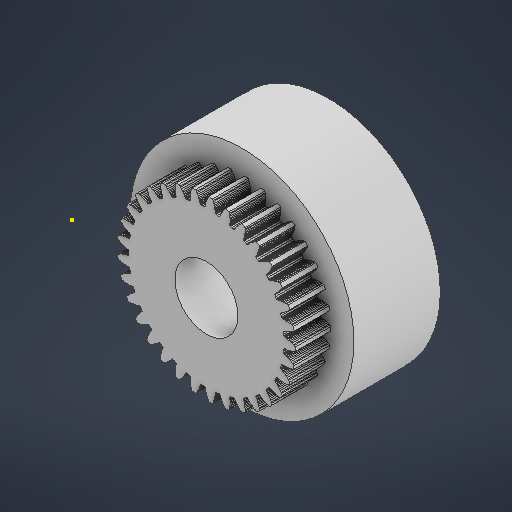
# Autodesk Inventor part: EngranajeRueda
Saved by Autodesk Inventor 2027 (Build 310192060, 192F)
## iProperties
Created: 2026-08-10
Part Number: EngranajeRueda
Material: Generic
Document SubType Name: Modeling
Designer: Administrator
Density: 1 g/cm^3
Appearance: Default
Author: Administrator
Autodesk Inventor part; units mm, degrees
(part 1 of 3)
ref_plane "YZ Plane" through (0, 0, 0) normal (1, 0, 0) x (0, 1, 0)
ref_plane "XZ Plane" through (0, 0, 0) normal (0, 1, 0) x (-1, 0, 0)
ref_plane "XY Plane" through (0, 0, 0) normal (0, 0, 1) x (1, 0, 0)
sketch "Sketch1" plane through (0, 0, 0) normal (0, 0, 1) x (1, 0, 0)
  point P0 (0, 0)
sketch "Sketch2" plane through (0, 0, 0) normal (0, 0, 1) x (1, 0, 0)
  circle A0 centre (13.25, 0) radius 4
  circle A1 centre (13.25, 0) radius 4
  line L0 (0, -0.275) -> (0, 0.275)
  line L1 (-0.275, 0) -> (0.275, 0)
  line L2 (0, -0.275) -> (0, 0.275)
  line L3 (-0.275, 0) -> (0.275, 0)
  line L4 (4.9115, -2.1897) -> (4.9704, -2.1401)
  line L5 (4.9704, -2.1401) -> (5.0843, -2.0503)
  line L6 (5.0843, -2.0503) -> (5.1901, -1.9738)
  line L7 (5.1901, -1.9738) -> (5.2873, -1.9095)
  line L8 (5.2873, -1.9095) -> (5.3762, -1.8559)
  line L9 (5.3762, -1.8559) -> (5.4548, -1.8129)
  line L10 (5.4548, -1.8129) -> (5.5252, -1.7781)
  line L11 (5.5252, -1.7781) -> (5.5804, -1.7537)
  line L12 (5.5804, -1.7537) -> (5.6607, -1.7208)
  line L13 (5.6607, -1.7208) -> (5.6881, -1.7069)
  line L14 (5.6881, -1.7069) -> (5.7116, -1.6927)
  line L15 (5.7116, -1.6927) -> (5.7313, -1.6783)
  line L16 (5.7313, -1.6783) -> (5.747, -1.6639)
  line L17 (5.747, -1.6639) -> (5.7588, -1.6496)
  line L18 (5.7588, -1.6496) -> (5.7667, -1.6357)
  line L19 (5.7667, -1.6357) -> (5.7708, -1.6222)
  line L20 (5.7708, -1.6222) -> (5.7711, -1.6094)
  line L21 (5.7711, -1.6094) -> (5.7661, -1.5858)
  line L22 (5.7661, -1.5858) -> (5.7382, -1.4478)
  line L23 (5.7382, -1.4478) -> (5.7128, -1.3093)
  line L24 (5.7128, -1.3093) -> (5.7087, -1.2856)
  line L25 (5.7087, -1.2856) -> (5.7036, -1.2737)
  line L26 (5.7036, -1.2737) -> (5.6948, -1.2627)
  line L27 (5.6948, -1.2627) -> (5.6823, -1.2527)
  line L28 (5.6823, -1.2527) -> (5.666, -1.2439)
  line L29 (5.666, -1.2439) -> (5.6461, -1.2364)
  line L30 (5.6461, -1.2364) -> (5.6225, -1.2303)
  line L31 (5.6225, -1.2303) -> (5.5954, -1.2258)
  line L32 (5.5954, -1.2258) -> (5.5648, -1.2231)
  line L33 (5.5648, -1.2231) -> (5.478, -1.2224)
  line L34 (5.478, -1.2224) -> (5.4177, -1.2203)
  line L35 (5.4177, -1.2203) -> (5.3394, -1.2142)
  line L36 (5.3394, -1.2142) -> (5.2505, -1.2034)
  line L37 (5.2505, -1.2034) -> (5.148, -1.1867)
  line L38 (5.148, -1.1867) -> (5.0338, -1.1631)
  line L39 (5.0338, -1.1631) -> (4.9072, -1.1315)
  line L40 (4.9072, -1.1315) -> (4.7681, -1.0904)
  line L41 (4.7681, -1.0904) -> (4.695, -1.0663)
  line L42 (4.695, -1.0663) -> (4.5593, -1.0171)
  arc A2 (4.5239, -0.646) -> (4.5593, -1.0171) centre (13.25, 0) ccw
  line L43 (4.5239, -0.646) -> (4.6478, -0.572)
  line L44 (4.6478, -0.572) -> (4.715, -0.5346)
  line L45 (4.715, -0.5346) -> (4.8439, -0.4679)
  line L46 (4.8439, -0.4679) -> (4.9622, -0.4128)
  line L47 (4.9622, -0.4128) -> (5.0698, -0.368)
  line L48 (5.0698, -0.368) -> (5.1673, -0.3322)
  line L49 (5.1673, -0.3322) -> (5.2526, -0.3049)
  line L50 (5.2526, -0.3049) -> (5.3283, -0.2841)
  line L51 (5.3283, -0.2841) -> (5.3871, -0.2705)
  line L52 (5.3871, -0.2705) -> (5.4722, -0.2535)
  line L53 (5.4722, -0.2535) -> (5.5017, -0.245)
  line L54 (5.5017, -0.245) -> (5.5275, -0.2354)
  line L55 (5.5275, -0.2354) -> (5.5495, -0.225)
  line L56 (5.5495, -0.225) -> (5.5677, -0.2139)
  line L57 (5.5677, -0.2139) -> (5.582, -0.2021)
  line L58 (5.582, -0.2021) -> (5.5924, -0.1899)
  line L59 (5.5924, -0.1899) -> (5.599, -0.1775)
  line L60 (5.599, -0.1775) -> (5.6017, -0.1649)
  line L61 (5.6017, -0.1649) -> (5.6013, -0.1408)
  line L62 (5.6013, -0.1408) -> (5.6, 0)
  line L63 (5.6, 0) -> (5.6013, 0.1408)
  line L64 (5.6013, 0.1408) -> (5.6017, 0.1649)
  line L65 (5.6017, 0.1649) -> (5.599, 0.1775)
  line L66 (5.599, 0.1775) -> (5.5924, 0.1899)
  line L67 (5.5924, 0.1899) -> (5.582, 0.2021)
  line L68 (5.582, 0.2021) -> (5.5677, 0.2139)
  line L69 (5.5677, 0.2139) -> (5.5495, 0.225)
  line L70 (5.5495, 0.225) -> (5.5275, 0.2354)
  line L71 (5.5275, 0.2354) -> (5.5017, 0.245)
  line L72 (5.5017, 0.245) -> (5.4722, 0.2535)
  line L73 (5.4722, 0.2535) -> (5.3871, 0.2705)
  line L74 (5.3871, 0.2705) -> (5.3283, 0.2841)
  line L75 (5.3283, 0.2841) -> (5.2526, 0.3049)
  line L76 (5.2526, 0.3049) -> (5.1673, 0.3322)
  line L77 (5.1673, 0.3322) -> (5.0698, 0.368)
  line L78 (5.0698, 0.368) -> (4.9622, 0.4128)
  line L79 (4.9622, 0.4128) -> (4.8439, 0.4679)
  line L80 (4.8439, 0.4679) -> (4.715, 0.5346)
  line L81 (4.715, 0.5346) -> (4.6478, 0.572)
  line L82 (4.6478, 0.572) -> (4.5239, 0.646)
  arc A3 (4.5593, 1.0171) -> (4.5239, 0.646) centre (13.25, 0) ccw
  line L83 (4.5593, 1.0171) -> (4.695, 1.0663)
  line L84 (4.695, 1.0663) -> (4.7681, 1.0904)
  line L85 (4.7681, 1.0904) -> (4.9072, 1.1315)
  line L86 (4.9072, 1.1315) -> (5.0338, 1.1631)
  line L87 (5.0338, 1.1631) -> (5.148, 1.1867)
  line L88 (5.148, 1.1867) -> (5.2505, 1.2034)
  line L89 (5.2505, 1.2034) -> (5.3394, 1.2142)
  line L90 (5.3394, 1.2142) -> (5.4177, 1.2203)
  line L91 (5.4177, 1.2203) -> (5.478, 1.2224)
  line L92 (5.478, 1.2224) -> (5.5648, 1.2231)
  line L93 (5.5648, 1.2231) -> (5.5954, 1.2258)
  line L94 (5.5954, 1.2258) -> (5.6225, 1.2303)
  line L95 (5.6225, 1.2303) -> (5.6461, 1.2364)
  line L96 (5.6461, 1.2364) -> (5.666, 1.2439)
  line L97 (5.666, 1.2439) -> (5.6823, 1.2527)
  line L98 (5.6823, 1.2527) -> (5.6948, 1.2627)
  line L99 (5.6948, 1.2627) -> (5.7036, 1.2737)
  line L100 (5.7036, 1.2737) -> (5.7087, 1.2856)
  line L101 (5.7087, 1.2856) -> (5.7128, 1.3093)
  line L102 (5.7128, 1.3093) -> (5.7382, 1.4478)
  line L103 (5.7382, 1.4478) -> (5.7661, 1.5858)
  line L104 (5.7661, 1.5858) -> (5.7711, 1.6094)
  line L105 (5.7711, 1.6094) -> (5.7708, 1.6222)
  line L106 (5.7708, 1.6222) -> (5.7667, 1.6357)
  line L107 (5.7667, 1.6357) -> (5.7588, 1.6496)
  line L108 (5.7588, 1.6496) -> (5.747, 1.6639)
  line L109 (5.747, 1.6639) -> (5.7313, 1.6783)
  line L110 (5.7313, 1.6783) -> (5.7116, 1.6927)
  line L111 (5.7116, 1.6927) -> (5.6881, 1.7069)
  line L112 (5.6881, 1.7069) -> (5.6607, 1.7208)
  line L113 (5.6607, 1.7208) -> (5.5804, 1.7537)
  line L114 (5.5804, 1.7537) -> (5.5252, 1.7781)
  line L115 (5.5252, 1.7781) -> (5.4548, 1.8129)
  line L116 (5.4548, 1.8129) -> (5.3762, 1.8559)
  line L117 (5.3762, 1.8559) -> (5.2873, 1.9095)
  line L118 (5.2873, 1.9095) -> (5.1901, 1.9738)
  line L119 (5.1901, 1.9738) -> (5.0843, 2.0503)
  line L120 (5.0843, 2.0503) -> (4.9704, 2.1401)
  line L121 (4.9704, 2.1401) -> (4.9115, 2.1897)
  line L122 (4.9115, 2.1897) -> (4.8038, 2.2858)
  arc A4 (4.9089, 2.6434) -> (4.8038, 2.2858) centre (13.25, 0) ccw
  line L123 (4.9089, 2.6434) -> (5.0514, 2.666)
  line L124 (5.0514, 2.666) -> (5.1277, 2.6759)
  line L125 (5.1277, 2.6759) -> (5.2721, 2.6899)
  line L126 (5.2721, 2.6899) -> (5.4024, 2.697)
  line L127 (5.4024, 2.697) -> (5.519, 2.6986)
  line L128 (5.519, 2.6986) -> (5.6228, 2.6956)
  line L129 (5.6228, 2.6956) -> (5.7121, 2.6893)
  line L130 (5.7121, 2.6893) -> (5.7902, 2.6805)
  line L131 (5.7902, 2.6805) -> (5.8498, 2.6712)
  line L132 (5.8498, 2.6712) -> (5.9351, 2.6554)
  line L133 (5.9351, 2.6554) -> (5.9657, 2.6523)
  line L134 (5.9657, 2.6523) -> (5.9932, 2.6516)
  line L135 (5.9932, 2.6516) -> (6.0175, 2.6531)
  line L136 (6.0175, 2.6531) -> (6.0385, 2.6567)
  line L137 (6.0385, 2.6567) -> (6.0561, 2.6623)
  line L138 (6.0561, 2.6623) -> (6.0703, 2.6697)
  line L139 (6.0703, 2.6697) -> (6.0811, 2.6789)
  line L140 (6.0811, 2.6789) -> (6.0882, 2.6895)
  line L141 (6.0882, 2.6895) -> (6.0968, 2.712)
  line L142 (6.0968, 2.712) -> (6.148, 2.8432)
  line L143 (6.148, 2.8432) -> (6.2015, 2.9735)
  line L144 (6.2015, 2.9735) -> (6.2108, 2.9957)
  line L145 (6.2108, 2.9957) -> (6.213, 3.0083)
  line L146 (6.213, 3.0083) -> (6.2115, 3.0223)
  line L147 (6.2115, 3.0223) -> (6.2064, 3.0375)
  line L148 (6.2064, 3.0375) -> (6.1974, 3.0538)
  line L149 (6.1974, 3.0538) -> (6.1847, 3.0709)
  line L150 (6.1847, 3.0709) -> (6.1682, 3.0887)
  line L151 (6.1682, 3.0887) -> (6.1478, 3.1072)
  line L152 (6.1478, 3.1072) -> (6.1235, 3.126)
  line L153 (6.1235, 3.126) -> (6.0508, 3.1735)
  line L154 (6.0508, 3.1735) -> (6.0013, 3.2079)
  line L155 (6.0013, 3.2079) -> (5.9387, 3.2554)
  line L156 (5.9387, 3.2554) -> (5.8698, 3.3125)
  line L157 (5.8698, 3.3125) -> (5.7926, 3.3819)
  line L158 (5.7926, 3.3819) -> (5.7093, 3.4635)
  line L159 (5.7093, 3.4635) -> (5.6199, 3.5586)
  line L160 (5.6199, 3.5586) -> (5.5251, 3.6684)
  line L161 (5.5251, 3.6684) -> (5.4766, 3.7282)
  line L162 (5.4766, 3.7282) -> (5.3891, 3.8429)
  arc A5 (5.5599, 4.1742) -> (5.3891, 3.8429) centre (13.25, 0) ccw
  line L163 (5.5599, 4.1742) -> (5.7041, 4.1695)
  line L164 (5.7041, 4.1695) -> (5.7809, 4.1647)
  line L165 (5.7809, 4.1647) -> (5.9254, 4.1511)
  line L166 (5.9254, 4.1511) -> (6.0547, 4.1335)
  line L167 (6.0547, 4.1335) -> (6.1694, 4.1129)
  line L168 (6.1694, 4.1129) -> (6.2708, 4.0904)
  line L169 (6.2708, 4.0904) -> (6.3573, 4.0673)
  line L170 (6.3573, 4.0673) -> (6.4323, 4.0438)
  line L171 (6.4323, 4.0438) -> (6.489, 4.0235)
  line L172 (6.489, 4.0235) -> (6.5698, 3.9918)
  line L173 (6.5698, 3.9918) -> (6.5993, 3.9829)
  line L174 (6.5993, 3.9829) -> (6.6262, 3.977)
  line L175 (6.6262, 3.977) -> (6.6503, 3.9739)
  line L176 (6.6503, 3.9739) -> (6.6716, 3.9735)
  line L177 (6.6716, 3.9735) -> (6.69, 3.9756)
  line L178 (6.69, 3.9756) -> (6.7053, 3.9802)
  line L179 (6.7053, 3.9802) -> (6.7176, 3.9872)
  line L180 (6.7176, 3.9872) -> (6.7267, 3.9963)
  line L181 (6.7267, 3.9963) -> (6.7394, 4.0168)
  line L182 (6.7394, 4.0168) -> (6.8144, 4.1359)
  line L183 (6.8144, 4.1359) -> (6.8916, 4.2537)
  line L184 (6.8916, 4.2537) -> (6.9049, 4.2737)
  line L185 (6.9049, 4.2737) -> (6.9095, 4.2857)
  line L186 (6.9095, 4.2857) -> (6.9107, 4.2998)
  line L187 (6.9107, 4.2998) -> (6.9085, 4.3157)
  line L188 (6.9085, 4.3157) -> (6.9028, 4.3333)
  line L189 (6.9028, 4.3333) -> (6.8936, 4.3525)
  line L190 (6.8936, 4.3525) -> (6.8807, 4.3732)
  line L191 (6.8807, 4.3732) -> (6.8642, 4.3951)
  line L192 (6.8642, 4.3951) -> (6.8439, 4.4182)
  line L193 (6.8439, 4.4182) -> (6.7815, 4.4786)
  line L194 (6.7815, 4.4786) -> (6.7394, 4.5218)
  line L195 (6.7394, 4.5218) -> (6.6869, 4.5802)
  line L196 (6.6869, 4.5802) -> (6.63, 4.6493)
  line L197 (6.63, 4.6493) -> (6.5674, 4.7321)
  line L198 (6.5674, 4.7321) -> (6.501, 4.828)
  line L199 (6.501, 4.828) -> (6.4313, 4.9383)
  line L200 (6.4313, 4.9383) -> (6.3589, 5.064)
  line L201 (6.3589, 5.064) -> (6.3226, 5.1319)
  line L202 (6.3226, 5.1319) -> (6.2584, 5.2612)
  arc A6 (6.4888, 5.5542) -> (6.2584, 5.2612) centre (13.25, 0) ccw
  line L203 (6.4888, 5.5542) -> (6.6295, 5.5222)
  line L204 (6.6295, 5.5222) -> (6.7041, 5.5029)
  line L205 (6.7041, 5.5029) -> (6.8433, 5.4623)
  line L206 (6.8433, 5.4623) -> (6.967, 5.4205)
  line L207 (6.967, 5.4205) -> (7.0758, 5.3786)
  line L208 (7.0758, 5.3786) -> (7.171, 5.3373)
  line L209 (7.171, 5.3373) -> (7.2516, 5.2982)
  line L210 (7.2516, 5.2982) -> (7.3208, 5.261)
  line L211 (7.3208, 5.261) -> (7.3727, 5.2303)
  line L212 (7.3727, 5.2303) -> (7.446, 5.1839)
  line L213 (7.446, 5.1839) -> (7.4733, 5.1696)
  line L214 (7.4733, 5.1696) -> (7.4985, 5.1587)
  line L215 (7.4985, 5.1587) -> (7.5216, 5.1511)
  line L216 (7.5216, 5.1511) -> (7.5424, 5.1466)
  line L217 (7.5424, 5.1466) -> (7.5609, 5.1453)
  line L218 (7.5609, 5.1453) -> (7.5769, 5.1469)
  line L219 (7.5769, 5.1469) -> (7.5902, 5.1514)
  line L220 (7.5902, 5.1514) -> (7.6008, 5.1586)
  line L221 (7.6008, 5.1586) -> (7.6172, 5.1763)
  line L222 (7.6172, 5.1763) -> (7.7134, 5.2791)
  line L223 (7.7134, 5.2791) -> (7.8115, 5.3801)
  line L224 (7.8115, 5.3801) -> (7.8284, 5.3973)
  line L225 (7.8284, 5.3973) -> (7.8352, 5.4082)
  line L226 (7.8352, 5.4082) -> (7.839, 5.4218)
  line L227 (7.839, 5.4218) -> (7.8399, 5.4378)
  line L228 (7.8399, 5.4378) -> (7.8376, 5.4562)
  line L229 (7.8376, 5.4562) -> (7.8322, 5.4768)
  line L230 (7.8322, 5.4768) -> (7.8235, 5.4995)
  line L231 (7.8235, 5.4995) -> (7.8114, 5.5242)
  line L232 (7.8114, 5.5242) -> (7.7958, 5.5508)
  line L233 (7.7958, 5.5508) -> (7.746, 5.6218)
  line L234 (7.746, 5.6218) -> (7.7128, 5.6722)
  line L235 (7.7128, 5.6722) -> (7.6724, 5.7395)
  line L236 (7.6724, 5.7395) -> (7.6295, 5.8181)
  line L237 (7.6295, 5.8181) -> (7.5837, 5.9113)
  line L238 (7.5837, 5.9113) -> (7.5367, 6.018)
  line L239 (7.5367, 6.018) -> (7.4891, 6.1395)
  line L240 (7.4891, 6.1395) -> (7.4418, 6.2767)
  line L241 (7.4418, 6.2767) -> (7.4191, 6.3502)
  line L242 (7.4191, 6.3502) -> (7.3804, 6.4893)
  arc A7 (7.6621, 6.7334) -> (7.3804, 6.4893) centre (13.25, 0) ccw
  line L243 (7.6621, 6.7334) -> (7.7943, 6.6753)
  line L244 (7.7943, 6.6753) -> (7.8638, 6.6423)
  line L245 (7.8638, 6.6423) -> (7.9928, 6.576)
  line L246 (7.9928, 6.576) -> (8.1063, 6.5116)
  line L247 (8.1063, 6.5116) -> (8.2052, 6.4499)
  line L248 (8.2052, 6.4499) -> (8.291, 6.3913)
  line L249 (8.291, 6.3913) -> (8.3627, 6.3377)
  line L250 (8.3627, 6.3377) -> (8.4236, 6.2881)
  line L251 (8.4236, 6.2881) -> (8.4687, 6.248)
  line L252 (8.4687, 6.248) -> (8.532, 6.1886)
  line L253 (8.532, 6.1886) -> (8.556, 6.1694)
  line L254 (8.556, 6.1694) -> (8.5787, 6.154)
  line L255 (8.5787, 6.154) -> (8.6, 6.1421)
  line L256 (8.6, 6.1421) -> (8.6196, 6.1338)
  line L257 (8.6196, 6.1338) -> (8.6375, 6.129)
  line L258 (8.6375, 6.129) -> (8.6535, 6.1275)
  line L259 (8.6535, 6.1275) -> (8.6674, 6.1294)
  line L260 (8.6674, 6.1294) -> (8.6792, 6.1345)
  line L261 (8.6792, 6.1345) -> (8.6986, 6.1488)
  line L262 (8.6986, 6.1488) -> (8.8126, 6.2315)
  line L263 (8.8126, 6.2315) -> (8.928, 6.3121)
  line L264 (8.928, 6.3121) -> (8.9478, 6.3258)
  line L265 (8.9478, 6.3258) -> (8.9565, 6.3353)
  line L266 (8.9565, 6.3353) -> (8.9629, 6.3479)
  line L267 (8.9629, 6.3479) -> (8.9667, 6.3634)
  line L268 (8.9667, 6.3634) -> (8.968, 6.3819)
  line L269 (8.968, 6.3819) -> (8.9666, 6.4032)
  line L270 (8.9666, 6.4032) -> (8.9623, 6.4271)
  line L271 (8.9623, 6.4271) -> (8.9551, 6.4536)
  line L272 (8.9551, 6.4536) -> (8.9449, 6.4827)
  line L273 (8.9449, 6.4827) -> (8.9094, 6.5619)
  line L274 (8.9094, 6.5619) -> (8.8863, 6.6176)
  line L275 (8.8863, 6.6176) -> (8.8594, 6.6914)
  line L276 (8.8594, 6.6914) -> (8.8322, 6.7767)
  line L277 (8.8322, 6.7767) -> (8.8048, 6.8769)
  line L278 (8.8048, 6.8769) -> (8.7788, 6.9905)
  line L279 (8.7788, 6.9905) -> (8.7551, 7.1188)
  line L280 (8.7551, 7.1188) -> (8.7347, 7.2624)
  line L281 (8.7347, 7.2624) -> (8.7262, 7.339)
  line L282 (8.7262, 7.339) -> (8.7146, 7.4828)
  arc A8 (9.0374, 7.6692) -> (8.7146, 7.4828) centre (13.25, 0) ccw
  line L283 (9.0374, 7.6692) -> (9.1562, 7.5872)
  line L284 (9.1562, 7.5872) -> (9.2182, 7.5416)
  line L285 (9.2182, 7.5416) -> (9.3324, 7.4521)
  line L286 (9.3324, 7.4521) -> (9.4316, 7.3674)
  line L287 (9.4316, 7.3674) -> (9.5171, 7.2881)
  line L288 (9.5171, 7.2881) -> (9.5901, 7.2143)
  line L289 (9.5901, 7.2143) -> (9.6504, 7.1481)
  line L290 (9.6504, 7.1481) -> (9.7008, 7.0878)
  line L291 (9.7008, 7.0878) -> (9.7376, 7.04)
  line L292 (9.7376, 7.04) -> (9.7884, 6.9697)
  line L293 (9.7884, 6.9697) -> (9.8084, 6.9463)
  line L294 (9.8084, 6.9463) -> (9.8278, 6.9268)
  line L295 (9.8278, 6.9268) -> (9.8464, 6.9111)
  line L296 (9.8464, 6.9111) -> (9.8641, 6.8993)
  line L297 (9.8641, 6.8993) -> (9.8807, 6.8911)
  line L298 (9.8807, 6.8911) -> (9.8962, 6.8867)
  line L299 (9.8962, 6.8867) -> (9.9102, 6.8859)
  line L300 (9.9102, 6.8859) -> (9.9228, 6.8887)
  line L301 (9.9228, 6.8887) -> (9.9445, 6.899)
  line L302 (9.9445, 6.899) -> (10.0721, 6.9587)
  line L303 (10.0721, 6.9587) -> (10.2007, 7.016)
  line L304 (10.2007, 7.016) -> (10.2227, 7.0257)
  line L305 (10.2227, 7.0257) -> (10.2331, 7.0333)
  line L306 (10.2331, 7.0333) -> (10.2417, 7.0445)
  line L307 (10.2417, 7.0445) -> (10.2484, 7.059)
  line L308 (10.2484, 7.059) -> (10.2532, 7.0769)
  line L309 (10.2532, 7.0769) -> (10.2558, 7.0981)
  line L310 (10.2558, 7.0981) -> (10.2561, 7.1224)
  line L311 (10.2561, 7.1224) -> (10.2541, 7.1498)
  line L312 (10.2541, 7.1498) -> (10.2495, 7.1803)
  line L313 (10.2495, 7.1803) -> (10.2297, 7.2647)
  line L314 (10.2297, 7.2647) -> (10.2176, 7.3238)
  line L315 (10.2176, 7.3238) -> (10.2051, 7.4014)
  line L316 (10.2051, 7.4014) -> (10.1945, 7.4903)
  line L317 (10.1945, 7.4903) -> (10.1866, 7.5938)
  line L318 (10.1866, 7.5938) -> (10.1826, 7.7103)
  line L319 (10.1826, 7.7103) -> (10.1836, 7.8409)
  line L320 (10.1836, 7.8409) -> (10.1907, 7.9857)
  line L321 (10.1907, 7.9857) -> (10.1969, 8.0625)
  line L322 (10.1969, 8.0625) -> (10.2127, 8.2059)
  arc A9 (10.5649, 8.3278) -> (10.2127, 8.2059) centre (13.25, 0) ccw
  line L323 (10.5649, 8.3278) -> (10.666, 8.2249)
  line L324 (10.666, 8.2249) -> (10.7183, 8.1683)
  line L325 (10.7183, 8.1683) -> (10.8135, 8.0589)
  line L326 (10.8135, 8.0589) -> (10.8949, 7.9569)
  line L327 (10.8949, 7.9569) -> (10.9638, 7.8628)
  line L328 (10.9638, 7.8628) -> (11.0216, 7.7765)
  line L329 (11.0216, 7.7765) -> (11.0683, 7.7001)
  line L330 (11.0683, 7.7001) -> (11.1063, 7.6314)
  line L331 (11.1063, 7.6314) -> (11.1334, 7.5775)
  line L332 (11.1334, 7.5775) -> (11.17, 7.4988)
  line L333 (11.17, 7.4988) -> (11.1852, 7.4721)
  line L334 (11.1852, 7.4721) -> (11.2005, 7.4493)
  line L335 (11.2005, 7.4493) -> (11.2159, 7.4304)
  line L336 (11.2159, 7.4304) -> (11.231, 7.4154)
  line L337 (11.231, 7.4154) -> (11.2458, 7.4042)
  line L338 (11.2458, 7.4042) -> (11.2601, 7.397)
  line L339 (11.2601, 7.397) -> (11.2737, 7.3935)
  line L340 (11.2737, 7.3935) -> (11.2866, 7.3939)
  line L341 (11.2866, 7.3939) -> (11.3099, 7.3999)
  line L342 (11.3099, 7.3999) -> (11.4464, 7.4344)
  line L343 (11.4464, 7.4344) -> (11.5836, 7.4663)
  line L344 (11.5836, 7.4663) -> (11.6071, 7.4716)
  line L345 (11.6071, 7.4716) -> (11.6187, 7.4772)
  line L346 (11.6187, 7.4772) -> (11.6292, 7.4865)
  line L347 (11.6292, 7.4865) -> (11.6386, 7.4995)
  line L348 (11.6386, 7.4995) -> (11.6467, 7.5162)
  line L349 (11.6467, 7.5162) -> (11.6532, 7.5365)
  line L350 (11.6532, 7.5365) -> (11.6582, 7.5603)
  line L351 (11.6582, 7.5603) -> (11.6614, 7.5876)
  line L352 (11.6614, 7.5876) -> (11.6626, 7.6183)
  line L353 (11.6626, 7.6183) -> (11.6591, 7.7051)
  line L354 (11.6591, 7.7051) -> (11.6584, 7.7654)
  line L355 (11.6584, 7.7654) -> (11.6608, 7.8439)
  line L356 (11.6608, 7.8439) -> (11.6673, 7.9332)
  line L357 (11.6673, 7.9332) -> (11.6791, 8.0364)
  line L358 (11.6791, 8.0364) -> (11.6972, 8.1515)
  line L359 (11.6972, 8.1515) -> (11.7229, 8.2795)
  line L360 (11.7229, 8.2795) -> (11.7573, 8.4204)
  line L361 (11.7573, 8.4204) -> (11.7779, 8.4946)
  line L362 (11.7779, 8.4946) -> (11.8205, 8.6324)
  arc A10 (12.1895, 8.6855) -> (11.8205, 8.6324) centre (13.25, 0) ccw
  line L363 (12.1895, 8.6855) -> (12.2693, 8.5652)
  line L364 (12.2693, 8.5652) -> (12.3099, 8.4999)
  line L365 (12.3099, 8.4999) -> (12.3827, 8.3744)
  line L366 (12.3827, 8.3744) -> (12.4433, 8.2588)
  line L367 (12.4433, 8.2588) -> (12.4931, 8.1534)
  line L368 (12.4931, 8.1534) -> (12.5336, 8.0577)
  line L369 (12.5336, 8.0577) -> (12.5649, 7.9739)
  line L370 (12.5649, 7.9739) -> (12.5893, 7.8992)
  line L371 (12.5893, 7.8992) -> (12.6057, 7.8412)
  line L372 (12.6057, 7.8412) -> (12.6267, 7.757)
  line L373 (12.6267, 7.757) -> (12.6366, 7.7278)
  line L374 (12.6366, 7.7278) -> (12.6474, 7.7025)
  line L375 (12.6474, 7.7025) -> (12.6588, 7.6811)
  line L376 (12.6588, 7.6811) -> (12.6708, 7.6635)
  line L377 (12.6708, 7.6635) -> (12.6833, 7.6497)
  line L378 (12.6833, 7.6497) -> (12.6959, 7.6399)
  line L379 (12.6959, 7.6399) -> (12.7087, 7.6339)
  line L380 (12.7087, 7.6339) -> (12.7214, 7.6318)
  line L381 (12.7214, 7.6318) -> (12.7454, 7.6334)
  line L382 (12.7454, 7.6334) -> (12.886, 7.6413)
  line L383 (12.886, 7.6413) -> (13.0267, 7.6468)
  line L384 (13.0267, 7.6468) -> (13.0508, 7.6475)
  line L385 (13.0508, 7.6475) -> (13.0632, 7.6508)
  line L386 (13.0632, 7.6508) -> (13.0753, 7.658)
  line L387 (13.0753, 7.658) -> (13.087, 7.669)
  line L388 (13.087, 7.669) -> (13.0981, 7.6838)
  line L389 (13.0981, 7.6838) -> (13.1084, 7.7025)
  line L390 (13.1084, 7.7025) -> (13.1177, 7.7249)
  line L391 (13.1177, 7.7249) -> (13.126, 7.7511)
  line L392 (13.126, 7.7511) -> (13.1331, 7.7811)
  line L393 (13.1331, 7.7811) -> (13.1461, 7.8669)
  line L394 (13.1461, 7.8669) -> (13.1568, 7.9262)
  line L395 (13.1568, 7.9262) -> (13.174, 8.0029)
  line L396 (13.174, 8.0029) -> (13.1973, 8.0893)
  line L397 (13.1973, 8.0893) -> (13.2284, 8.1884)
  line L398 (13.2284, 8.1884) -> (13.268, 8.2981)
  line L399 (13.268, 8.2981) -> (13.3174, 8.4189)
  line L400 (13.3174, 8.4189) -> (13.3778, 8.5507)
  line L401 (13.3778, 8.5507) -> (13.4121, 8.6197)
  line L402 (13.4121, 8.6197) -> (13.4801, 8.747)
  arc A11 (13.8524, 8.7292) -> (13.4801, 8.747) centre (13.25, 0) ccw
  line L403 (13.8524, 8.7292) -> (13.908, 8.5961)
  line L404 (13.908, 8.5961) -> (13.9355, 8.5242)
  line L405 (13.9355, 8.5242) -> (13.9832, 8.3872)
  line L406 (13.9832, 8.3872) -> (14.0209, 8.2622)
  line L407 (14.0209, 8.2622) -> (14.0499, 8.1493)
  line L408 (14.0499, 8.1493) -> (14.0714, 8.0477)
  line L409 (14.0714, 8.0477) -> (14.0864, 7.9594)
  line L410 (14.0864, 7.9594) -> (14.0962, 7.8815)
  line L411 (14.0962, 7.8815) -> (14.1013, 7.8214)
  line L412 (14.1013, 7.8214) -> (14.106, 7.7347)
  line L413 (14.106, 7.7347) -> (14.1102, 7.7043)
  line L414 (14.1102, 7.7043) -> (14.116, 7.6774)
  line L415 (14.116, 7.6774) -> (14.1232, 7.6541)
  line L416 (14.1232, 7.6541) -> (14.1316, 7.6346)
  line L417 (14.1316, 7.6346) -> (14.1412, 7.6187)
  line L418 (14.1412, 7.6187) -> (14.1518, 7.6067)
  line L419 (14.1518, 7.6067) -> (14.1632, 7.5984)
  line L420 (14.1632, 7.5984) -> (14.1753, 7.594)
  line L421 (14.1753, 7.594) -> (14.1992, 7.5909)
  line L422 (14.1992, 7.5909) -> (14.3387, 7.5721)
  line L423 (14.3387, 7.5721) -> (14.4779, 7.5508)
  line L424 (14.4779, 7.5508) -> (14.5017, 7.547)
  line L425 (14.5017, 7.547) -> (14.5145, 7.5479)
  line L426 (14.5145, 7.5479) -> (14.5278, 7.5526)
  line L427 (14.5278, 7.5526) -> (14.5413, 7.5612)
  line L428 (14.5413, 7.5612) -> (14.555, 7.5737)
  line L429 (14.555, 7.5737) -> (14.5686, 7.5901)
  line L430 (14.5686, 7.5901) -> (14.5821, 7.6104)
  line L431 (14.5821, 7.6104) -> (14.5952, 7.6345)
  line L432 (14.5952, 7.6345) -> (14.6078, 7.6626)
  line L433 (14.6078, 7.6626) -> (14.6368, 7.7444)
  line L434 (14.6368, 7.7444) -> (14.6585, 7.8006)
  line L435 (14.6585, 7.8006) -> (14.6899, 7.8727)
  line L436 (14.6899, 7.8727) -> (14.7291, 7.9531)
  line L437 (14.7291, 7.9531) -> (14.7785, 8.0445)
  line L438 (14.7785, 8.0445) -> (14.8381, 8.1447)
  line L439 (14.8381, 8.1447) -> (14.9094, 8.254)
  line L440 (14.9094, 8.254) -> (14.9938, 8.372)
  line L441 (14.9938, 8.372) -> (15.0404, 8.4332)
  line L442 (15.0404, 8.4332) -> (15.1313, 8.5454)
  arc A12 (15.4935, 8.4575) -> (15.1313, 8.5454) centre (13.25, 0) ccw
  line L443 (15.4935, 8.4575) -> (15.5229, 8.3162)
  line L444 (15.5229, 8.3162) -> (15.5364, 8.2404)
  line L445 (15.5364, 8.2404) -> (15.5572, 8.0968)
  line L446 (15.5572, 8.0968) -> (15.5706, 7.967)
  line L447 (15.5706, 7.967) -> (15.5777, 7.8506)
  line L448 (15.5777, 7.8506) -> (15.5796, 7.7468)
  line L449 (15.5796, 7.7468) -> (15.5776, 7.6573)
  line L450 (15.5776, 7.6573) -> (15.5725, 7.5789)
  line L451 (15.5725, 7.5789) -> (15.5661, 7.519)
  line L452 (15.5661, 7.519) -> (15.5544, 7.433)
  line L453 (15.5544, 7.433) -> (15.5527, 7.4022)
  line L454 (15.5527, 7.4022) -> (15.5533, 7.3747)
  line L455 (15.5533, 7.3747) -> (15.5559, 7.3506)
  line L456 (15.5559, 7.3506) -> (15.5605, 7.3298)
  line L457 (15.5605, 7.3298) -> (15.567, 7.3124)
  line L458 (15.567, 7.3124) -> (15.5751, 7.2986)
  line L459 (15.5751, 7.2986) -> (15.5847, 7.2883)
  line L460 (15.5847, 7.2883) -> (15.5957, 7.2816)
  line L461 (15.5957, 7.2816) -> (15.6186, 7.2741)
  line L462 (15.6186, 7.2741) -> (15.7521, 7.2293)
  line L463 (15.7521, 7.2293) -> (15.8847, 7.182)
  line L464 (15.8847, 7.182) -> (15.9073, 7.1738)
  line L465 (15.9073, 7.1738) -> (15.9201, 7.1722)
  line L466 (15.9201, 7.1722) -> (15.934, 7.1743)
  line L467 (15.934, 7.1743) -> (15.949, 7.1802)
  line L468 (15.949, 7.1802) -> (15.9647, 7.1899)
  line L469 (15.9647, 7.1899) -> (15.9812, 7.2034)
  line L470 (15.9812, 7.2034) -> (15.9983, 7.2207)
  line L471 (15.9983, 7.2207) -> (16.0157, 7.242)
  line L472 (16.0157, 7.242) -> (16.0334, 7.2672)
  line L473 (16.0334, 7.2672) -> (16.0773, 7.342)
  line L474 (16.0773, 7.342) -> (16.1094, 7.3931)
  line L475 (16.1094, 7.3931) -> (16.1538, 7.4579)
  line L476 (16.1538, 7.4579) -> (16.2075, 7.5295)
  line L477 (16.2075, 7.5295) -> (16.2733, 7.6099)
  line L478 (16.2733, 7.6099) -> (16.3508, 7.697)
  line L479 (16.3508, 7.697) -> (16.4415, 7.7908)
  line L480 (16.4415, 7.7908) -> (16.5467, 7.8907)
  line L481 (16.5467, 7.8907) -> (16.6041, 7.942)
  line L482 (16.6041, 7.942) -> (16.7145, 8.0349)
  arc A13 (17.0536, 7.88) -> (16.7145, 8.0349) centre (13.25, 0) ccw
  line L483 (17.0536, 7.88) -> (17.0557, 7.7357)
  line L484 (17.0557, 7.7357) -> (17.0545, 7.6588)
  line L485 (17.0545, 7.6588) -> (17.0479, 7.5139)
  line L486 (17.0479, 7.5139) -> (17.0364, 7.3838)
  line L487 (17.0364, 7.3838) -> (17.0214, 7.2683)
  line L488 (17.0214, 7.2683) -> (17.0036, 7.1659)
  line L489 (17.0036, 7.1659) -> (16.9847, 7.0784)
  line L490 (16.9847, 7.0784) -> (16.9649, 7.0024)
  line L491 (16.9649, 7.0024) -> (16.9472, 6.9448)
  line L492 (16.9472, 6.9448) -> (16.9194, 6.8625)
  line L493 (16.9194, 6.8625) -> (16.912, 6.8327)
  line L494 (16.912, 6.8327) -> (16.9073, 6.8056)
  line L495 (16.9073, 6.8056) -> (16.9054, 6.7813)
  line L496 (16.9054, 6.7813) -> (16.906, 6.76)
  line L497 (16.906, 6.76) -> (16.909, 6.7418)
  line L498 (16.909, 6.7418) -> (16.9143, 6.7266)
  line L499 (16.9143, 6.7266) -> (16.9218, 6.7147)
  line L500 (16.9218, 6.7147) -> (16.9314, 6.7061)
  line L501 (16.9314, 6.7061) -> (16.9524, 6.6944)
  line L502 (16.9524, 6.6944) -> (17.075, 6.6251)
  line L503 (17.075, 6.6251) -> (17.1963, 6.5536)
  line L504 (17.1963, 6.5536) -> (17.217, 6.5412)
  line L505 (17.217, 6.5412) -> (17.2292, 6.5373)
  line L506 (17.2292, 6.5373) -> (17.2433, 6.5367)
  line L507 (17.2433, 6.5367) -> (17.259, 6.5397)
  line L508 (17.259, 6.5397) -> (17.2764, 6.5462)
  line L509 (17.2764, 6.5462) -> (17.2951, 6.5563)
  line L510 (17.2951, 6.5563) -> (17.3151, 6.5701)
  line L511 (17.3151, 6.5701) -> (17.3363, 6.5877)
  line L512 (17.3363, 6.5877) -> (17.3584, 6.6091)
  line L513 (17.3584, 6.6091) -> (17.4157, 6.6742)
  line L514 (17.4157, 6.6742) -> (17.4568, 6.7184)
  line L515 (17.4568, 6.7184) -> (17.5128, 6.7736)
  line L516 (17.5128, 6.7736) -> (17.5791, 6.8337)
  line L517 (17.5791, 6.8337) -> (17.6588, 6.9002)
  line L518 (17.6588, 6.9002) -> (17.7514, 6.9711)
  line L519 (17.7514, 6.9711) -> (17.8583, 7.046)
  line L520 (17.8583, 7.046) -> (17.9804, 7.1242)
  line L521 (17.9804, 7.1242) -> (18.0465, 7.1637)
  line L522 (18.0465, 7.1637) -> (18.1725, 7.234)
  arc A14 (18.4762, 7.0178) -> (18.1725, 7.234) centre (13.25, 0) ccw
  line L523 (18.4762, 7.0178) -> (18.4509, 6.8757)
  line L524 (18.4509, 6.8757) -> (18.4352, 6.8003)
  line L525 (18.4352, 6.8003) -> (18.4013, 6.6593)
  line L526 (18.4013, 6.6593) -> (18.3654, 6.5338)
  line L527 (18.3654, 6.5338) -> (18.3287, 6.4232)
  line L528 (18.3287, 6.4232) -> (18.292, 6.326)
  line L529 (18.292, 6.326) -> (18.2568, 6.2437)
  line L530 (18.2568, 6.2437) -> (18.2229, 6.1728)
  line L531 (18.2229, 6.1728) -> (18.1947, 6.1196)
  line L532 (18.1947, 6.1196) -> (18.1518, 6.0441)
  line L533 (18.1518, 6.0441) -> (18.1389, 6.0162)
  line L534 (18.1389, 6.0162) -> (18.1292, 5.9904)
  line L535 (18.1292, 5.9904) -> (18.1227, 5.967)
  line L536 (18.1227, 5.967) -> (18.1192, 5.946)
  line L537 (18.1192, 5.946) -> (18.1188, 5.9275)
  line L538 (18.1188, 5.9275) -> (18.1211, 5.9116)
  line L539 (18.1211, 5.9116) -> (18.1262, 5.8985)
  line L540 (18.1262, 5.8985) -> (18.134, 5.8882)
  line L541 (18.134, 5.8882) -> (18.1524, 5.8727)
  line L542 (18.1524, 5.8727) -> (18.2597, 5.7815)
  line L543 (18.2597, 5.7815) -> (18.3653, 5.6883)
  line L544 (18.3653, 5.6883) -> (18.3832, 5.6723)
  line L545 (18.3832, 5.6723) -> (18.3945, 5.6661)
  line L546 (18.3945, 5.6661) -> (18.4082, 5.6629)
  line L547 (18.4082, 5.6629) -> (18.4242, 5.6628)
  line L548 (18.4242, 5.6628) -> (18.4425, 5.6659)
  line L549 (18.4425, 5.6659) -> (18.4628, 5.6723)
  line L550 (18.4628, 5.6723) -> (18.4851, 5.6821)
  line L551 (18.4851, 5.6821) -> (18.5092, 5.6953)
  line L552 (18.5092, 5.6953) -> (18.5349, 5.7121)
  line L553 (18.5349, 5.7121) -> (18.6036, 5.7653)
  line L554 (18.6036, 5.7653) -> (18.6523, 5.8008)
  line L555 (18.6523, 5.8008) -> (18.7176, 5.8444)
  line L556 (18.7176, 5.8444) -> (18.7941, 5.8909)
  line L557 (18.7941, 5.8909) -> (18.885, 5.9411)
  line L558 (18.885, 5.9411) -> (18.9893, 5.9932)
  line L559 (18.9893, 5.9932) -> (19.1084, 6.0465)
  line L560 (19.1084, 6.0465) -> (19.2432, 6.1002)
  line L561 (19.2432, 6.1002) -> (19.3156, 6.1265)
  line L562 (19.3156, 6.1265) -> (19.4526, 6.1717)
  arc A15 (19.7098, 5.9019) -> (19.4526, 6.1717) centre (13.25, 0) ccw
  line L563 (19.7098, 5.9019) -> (19.6582, 5.7672)
  line L564 (19.6582, 5.7672) -> (19.6285, 5.6961)
  line L565 (19.6285, 5.6961) -> (19.5685, 5.5641)
  line L566 (19.5685, 5.5641) -> (19.5095, 5.4477)
  line L567 (19.5095, 5.4477) -> (19.4525, 5.3459)
  line L568 (19.4525, 5.3459) -> (19.3981, 5.2575)
  line L569 (19.3981, 5.2575) -> (19.348, 5.1833)
  line L570 (19.348, 5.1833) -> (19.3013, 5.1201)
  line L571 (19.3013, 5.1201) -> (19.2635, 5.0732)
  line L572 (19.2635, 5.0732) -> (19.2071, 5.0072)
  line L573 (19.2071, 5.0072) -> (19.1891, 4.9822)
  line L574 (19.1891, 4.9822) -> (19.1747, 4.9588)
  line L575 (19.1747, 4.9588) -> (19.1639, 4.937)
  line L576 (19.1639, 4.937) -> (19.1565, 4.917)
  line L577 (19.1565, 4.917) -> (19.1525, 4.8989)
  line L578 (19.1525, 4.8989) -> (19.1519, 4.8829)
  line L579 (19.1519, 4.8829) -> (19.1544, 4.869)
  line L580 (19.1544, 4.869) -> (19.1601, 4.8575)
  line L581 (19.1601, 4.8575) -> (19.1753, 4.8388)
  line L582 (19.1753, 4.8388) -> (19.2633, 4.7289)
  line L583 (19.2633, 4.7289) -> (19.3493, 4.6175)
  line L584 (19.3493, 4.6175) -> (19.3639, 4.5983)
  line L585 (19.3639, 4.5983) -> (19.3738, 4.5901)
  line L586 (19.3738, 4.5901) -> (19.3867, 4.5843)
  line L587 (19.3867, 4.5843) -> (19.4024, 4.5812)
  line L588 (19.4024, 4.5812) -> (19.4209, 4.5808)
  line L589 (19.4209, 4.5808) -> (19.4421, 4.5832)
  line L590 (19.4421, 4.5832) -> (19.4658, 4.5886)
  line L591 (19.4658, 4.5886) -> (19.492, 4.5971)
  line L592 (19.492, 4.5971) -> (19.5205, 4.6087)
  line L593 (19.5205, 4.6087) -> (19.5979, 4.6479)
  line L594 (19.5979, 4.6479) -> (19.6525, 4.6736)
  line L595 (19.6525, 4.6736) -> (19.7249, 4.7041)
  line L596 (19.7249, 4.7041) -> (19.8088, 4.7352)
  line L597 (19.8088, 4.7352) -> (19.9076, 4.7673)
  line L598 (19.9076, 4.7673) -> (20.0198, 4.7987)
  line L599 (20.0198, 4.7987) -> (20.1469, 4.8286)
  line L600 (20.1469, 4.8286) -> (20.2894, 4.8558)
  line L601 (20.2894, 4.8558) -> (20.3654, 4.8679)
  line L602 (20.3654, 4.8679) -> (20.5085, 4.8863)
  arc A16 (20.7101, 4.5727) -> (20.5085, 4.8863) centre (13.25, 0) ccw
  line L603 (20.7101, 4.5727) -> (20.6338, 4.4502)
  line L604 (20.6338, 4.4502) -> (20.5912, 4.3861)
  line L605 (20.5912, 4.3861) -> (20.5073, 4.2678)
  line L606 (20.5073, 4.2678) -> (20.4273, 4.1646)
  line L607 (20.4273, 4.1646) -> (20.3522, 4.0755)
  line L608 (20.3522, 4.0755) -> (20.2819, 3.999)
  line L609 (20.2819, 3.999) -> (20.2187, 3.9356)
  line L610 (20.2187, 3.9356) -> (20.1609, 3.8824)
  line L611 (20.1609, 3.8824) -> (20.1149, 3.8434)
  line L612 (20.1149, 3.8434) -> (20.0471, 3.7893)
  line L613 (20.0471, 3.7893) -> (20.0247, 3.7682)
  line L614 (20.0247, 3.7682) -> (20.0061, 3.7479)
  line L615 (20.0061, 3.7479) -> (19.9914, 3.7286)
  line L616 (19.9914, 3.7286) -> (19.9803, 3.7103)
  line L617 (19.9803, 3.7103) -> (19.973, 3.6933)
  line L618 (19.973, 3.6933) -> (19.9693, 3.6777)
  line L619 (19.9693, 3.6777) -> (19.9692, 3.6636)
  line L620 (19.9692, 3.6636) -> (19.9726, 3.6512)
  line L621 (19.9726, 3.6512) -> (19.9839, 3.63)
  line L622 (19.9839, 3.63) -> (20.0496, 3.5054)
  line L623 (20.0496, 3.5054) -> (20.113, 3.3797)
  line L624 (20.113, 3.3797) -> (20.1237, 3.3581)
  line L625 (20.1237, 3.3581) -> (20.1318, 3.3482)
  line L626 (20.1318, 3.3482) -> (20.1434, 3.3401)
  line L627 (20.1434, 3.3401) -> (20.1582, 3.3341)
  line L628 (20.1582, 3.3341) -> (20.1763, 3.3302)
  line L629 (20.1763, 3.3302) -> (20.1976, 3.3286)
  line L630 (20.1976, 3.3286) -> (20.2219, 3.3294)
  line L631 (20.2219, 3.3294) -> (20.2492, 3.3327)
  line L632 (20.2492, 3.3327) -> (20.2794, 3.3387)
  line L633 (20.2794, 3.3387) -> (20.3628, 3.3626)
  line L634 (20.3628, 3.3626) -> (20.4212, 3.3775)
  line L635 (20.4212, 3.3775) -> (20.4981, 3.3937)
  line L636 (20.4981, 3.3937) -> (20.5864, 3.4084)
  line L637 (20.5864, 3.4084) -> (20.6895, 3.4212)
  line L638 (20.6895, 3.4212) -> (20.8057, 3.4308)
  line L639 (20.8057, 3.4308) -> (20.9361, 3.4361)
  line L640 (20.9361, 3.4361) -> (21.0811, 3.4358)
  line L641 (21.0811, 3.4358) -> (21.1581, 3.4333)
  line L642 (21.1581, 3.4333) -> (21.3021, 3.4243)
  arc A17 (21.4406, 3.0783) -> (21.3021, 3.4243) centre (13.25, 0) ccw
  line L643 (21.4406, 3.0783) -> (21.3426, 2.9724)
  line L644 (21.3426, 2.9724) -> (21.2886, 2.9175)
  line L645 (21.2886, 2.9175) -> (21.1838, 2.8172)
  line L646 (21.1838, 2.8172) -> (21.0858, 2.731)
  line L647 (21.0858, 2.731) -> (20.9951, 2.6578)
  line L648 (20.9951, 2.6578) -> (20.9117, 2.5959)
  line L649 (20.9117, 2.5959) -> (20.8376, 2.5457)
  line L650 (20.8376, 2.5457) -> (20.7708, 2.5043)
  line L651 (20.7708, 2.5043) -> (20.7182, 2.4748)
  line L652 (20.7182, 2.4748) -> (20.6414, 2.4345)
  line L653 (20.6414, 2.4345) -> (20.6154, 2.418)
  line L654 (20.6154, 2.418) -> (20.5933, 2.4016)
  line L655 (20.5933, 2.4016) -> (20.5752, 2.3854)
  line L656 (20.5752, 2.3854) -> (20.5609, 2.3696)
  line L657 (20.5609, 2.3696) -> (20.5505, 2.3542)
  line L658 (20.5505, 2.3542) -> (20.5439, 2.3396)
  line L659 (20.5439, 2.3396) -> (20.5411, 2.3258)
  line L660 (20.5411, 2.3258) -> (20.5421, 2.313)
  line L661 (20.5421, 2.313) -> (20.5492, 2.29)
  line L662 (20.5492, 2.29) -> (20.5901, 2.1553)
  line L663 (20.5901, 2.1553) -> (20.6286, 2.0198)
  line L664 (20.6286, 2.0198) -> (20.635, 1.9966)
  line L665 (20.635, 1.9966) -> (20.6411, 1.9853)
  line L666 (20.6411, 1.9853) -> (20.6509, 1.9752)
  line L667 (20.6509, 1.9752) -> (20.6644, 1.9664)
  line L668 (20.6644, 1.9664) -> (20.6814, 1.9592)
  line L669 (20.6814, 1.9592) -> (20.702, 1.9536)
  line L670 (20.702, 1.9536) -> (20.726, 1.9498)
  line L671 (20.726, 1.9498) -> (20.7534, 1.9479)
  line L672 (20.7534, 1.9479) -> (20.7842, 1.9481)
  line L673 (20.7842, 1.9481) -> (20.8706, 1.9557)
  line L674 (20.8706, 1.9557) -> (20.9308, 1.9593)
  line L675 (20.9308, 1.9593) -> (21.0094, 1.9606)
  line L676 (21.0094, 1.9606) -> (21.0989, 1.9584)
  line L677 (21.0989, 1.9584) -> (21.2025, 1.9515)
  line L678 (21.2025, 1.9515) -> (21.3184, 1.9389)
  line L679 (21.3184, 1.9389) -> (21.4474, 1.9194)
  line L680 (21.4474, 1.9194) -> (21.5898, 1.8917)
  line L681 (21.5898, 1.8917) -> (21.6649, 1.8746)
  line L682 (21.6649, 1.8746) -> (21.8047, 1.8386)
  arc A18 (21.8752, 1.4726) -> (21.8047, 1.8386) centre (13.25, 0) ccw
  line L683 (21.8752, 1.4726) -> (21.7589, 1.3872)
  line L684 (21.7589, 1.3872) -> (21.6955, 1.3434)
  line L685 (21.6955, 1.3434) -> (21.5736, 1.2648)
  line L686 (21.5736, 1.2648) -> (21.461, 1.1987)
  line L687 (21.461, 1.1987) -> (21.3581, 1.1439)
  line L688 (21.3581, 1.1439) -> (21.2645, 1.099)
  line L689 (21.2645, 1.099) -> (21.1823, 1.0637)
  line L690 (21.1823, 1.0637) -> (21.1088, 1.0358)
  line L691 (21.1088, 1.0358) -> (21.0516, 1.0167)
  line L692 (21.0516, 1.0167) -> (20.9685, 0.9916)
  line L693 (20.9685, 0.9916) -> (20.9399, 0.9804)
  line L694 (20.9399, 0.9804) -> (20.9151, 0.9685)
  line L695 (20.9151, 0.9685) -> (20.8942, 0.956)
  line L696 (20.8942, 0.956) -> (20.8772, 0.9431)
  line L697 (20.8772, 0.9431) -> (20.8641, 0.9301)
  line L698 (20.8641, 0.9301) -> (20.8549, 0.917)
  line L699 (20.8549, 0.917) -> (20.8495, 0.9039)
  line L700 (20.8495, 0.9039) -> (20.848, 0.8912)
  line L701 (20.848, 0.8912) -> (20.8507, 0.8672)
  line L702 (20.8507, 0.8672) -> (20.8654, 0.7272)
  line L703 (20.8654, 0.7272) -> (20.8775, 0.5869)
  line L704 (20.8775, 0.5869) -> (20.8794, 0.5629)
  line L705 (20.8794, 0.5629) -> (20.8833, 0.5506)
  line L706 (20.8833, 0.5506) -> (20.891, 0.5389)
  line L707 (20.891, 0.5389) -> (20.9025, 0.5277)
  line L708 (20.9025, 0.5277) -> (20.9179, 0.5174)
  line L709 (20.9179, 0.5174) -> (20.937, 0.508)
  line L710 (20.937, 0.508) -> (20.9599, 0.4997)
  line L711 (20.9599, 0.4997) -> (20.9865, 0.4926)
  line L712 (20.9865, 0.4926) -> (21.0167, 0.487)
  line L713 (21.0167, 0.487) -> (21.103, 0.4781)
  line L714 (21.103, 0.4781) -> (21.1628, 0.4702)
  line L715 (21.1628, 0.4702) -> (21.2402, 0.4567)
  line L716 (21.2402, 0.4567) -> (21.3277, 0.4376)
  line L717 (21.3277, 0.4376) -> (21.4281, 0.4112)
  line L718 (21.4281, 0.4112) -> (21.5395, 0.3769)
  line L719 (21.5395, 0.3769) -> (21.6626, 0.3333)
  line L720 (21.6626, 0.3333) -> (21.7971, 0.2792)
  line L721 (21.7971, 0.2792) -> (21.8676, 0.2482)
  line L722 (21.8676, 0.2482) -> (21.998, 0.1864)
  arc A19 (21.998, -0.1864) -> (21.998, 0.1864) centre (13.25, 0) ccw
  line L723 (21.998, -0.1864) -> (21.8676, -0.2482)
  line L724 (21.8676, -0.2482) -> (21.7971, -0.2792)
  line L725 (21.7971, -0.2792) -> (21.6626, -0.3333)
  line L726 (21.6626, -0.3333) -> (21.5395, -0.3769)
  line L727 (21.5395, -0.3769) -> (21.4281, -0.4112)
  line L728 (21.4281, -0.4112) -> (21.3277, -0.4376)
  line L729 (21.3277, -0.4376) -> (21.2402, -0.4567)
  line L730 (21.2402, -0.4567) -> (21.1628, -0.4702)
  line L731 (21.1628, -0.4702) -> (21.103, -0.4781)
  line L732 (21.103, -0.4781) -> (21.0167, -0.487)
  line L733 (21.0167, -0.487) -> (20.9865, -0.4926)
  line L734 (20.9865, -0.4926) -> (20.9599, -0.4997)
  line L735 (20.9599, -0.4997) -> (20.937, -0.508)
  line L736 (20.937, -0.508) -> (20.9179, -0.5174)
  line L737 (20.9179, -0.5174) -> (20.9025, -0.5277)
  line L738 (20.9025, -0.5277) -> (20.891, -0.5389)
  line L739 (20.891, -0.5389) -> (20.8833, -0.5506)
  line L740 (20.8833, -0.5506) -> (20.8794, -0.5629)
  line L741 (20.8794, -0.5629) -> (20.8775, -0.5869)
  line L742 (20.8775, -0.5869) -> (20.8654, -0.7272)
  line L743 (20.8654, -0.7272) -> (20.8507, -0.8672)
  line L744 (20.8507, -0.8672) -> (20.848, -0.8912)
  line L745 (20.848, -0.8912) -> (20.8495, -0.9039)
  line L746 (20.8495, -0.9039) -> (20.8549, -0.917)
  line L747 (20.8549, -0.917) -> (20.8641, -0.9301)
  line L748 (20.8641, -0.9301) -> (20.8772, -0.9431)
  line L749 (20.8772, -0.9431) -> (20.8942, -0.956)
  line L750 (20.8942, -0.956) -> (20.9151, -0.9685)
  line L751 (20.9151, -0.9685) -> (20.9399, -0.9804)
  line L752 (20.9399, -0.9804) -> (20.9685, -0.9916)
  line L753 (20.9685, -0.9916) -> (21.0516, -1.0167)
  line L754 (21.0516, -1.0167) -> (21.1088, -1.0358)
  line L755 (21.1088, -1.0358) -> (21.1823, -1.0637)
  line L756 (21.1823, -1.0637) -> (21.2645, -1.099)
  line L757 (21.2645, -1.099) -> (21.3581, -1.1439)
  line L758 (21.3581, -1.1439) -> (21.461, -1.1987)
  line L759 (21.461, -1.1987) -> (21.5736, -1.2648)
  line L760 (21.5736, -1.2648) -> (21.6955, -1.3434)
  line L761 (21.6955, -1.3434) -> (21.7589, -1.3872)
  line L762 (21.7589, -1.3872) -> (21.8752, -1.4726)
  arc A20 (21.8047, -1.8386) -> (21.8752, -1.4726) centre (13.25, 0) ccw
  line L763 (21.8047, -1.8386) -> (21.6649, -1.8746)
  line L764 (21.6649, -1.8746) -> (21.5898, -1.8917)
  line L765 (21.5898, -1.8917) -> (21.4474, -1.9194)
  line L766 (21.4474, -1.9194) -> (21.3184, -1.9389)
  line L767 (21.3184, -1.9389) -> (21.2025, -1.9515)
  line L768 (21.2025, -1.9515) -> (21.0989, -1.9584)
  line L769 (21.0989, -1.9584) -> (21.0094, -1.9606)
  line L770 (21.0094, -1.9606) -> (20.9308, -1.9593)
  line L771 (20.9308, -1.9593) -> (20.8706, -1.9557)
  line L772 (20.8706, -1.9557) -> (20.7842, -1.9481)
  line L773 (20.7842, -1.9481) -> (20.7534, -1.9479)
  line L774 (20.7534, -1.9479) -> (20.726, -1.9498)
  line L775 (20.726, -1.9498) -> (20.702, -1.9536)
  line L776 (20.702, -1.9536) -> (20.6814, -1.9592)
  line L777 (20.6814, -1.9592) -> (20.6644, -1.9664)
  line L778 (20.6644, -1.9664) -> (20.6509, -1.9752)
  line L779 (20.6509, -1.9752) -> (20.6411, -1.9853)
  line L780 (20.6411, -1.9853) -> (20.635, -1.9966)
  line L781 (20.635, -1.9966) -> (20.6286, -2.0198)
  line L782 (20.6286, -2.0198) -> (20.5901, -2.1553)
  line L783 (20.5901, -2.1553) -> (20.5492, -2.29)
  line L784 (20.5492, -2.29) -> (20.5421, -2.313)
  line L785 (20.5421, -2.313) -> (20.5411, -2.3258)
  line L786 (20.5411, -2.3258) -> (20.5439, -2.3396)
  line L787 (20.5439, -2.3396) -> (20.5505, -2.3542)
  line L788 (20.5505, -2.3542) -> (20.5609, -2.3696)
  line L789 (20.5609, -2.3696) -> (20.5752, -2.3854)
  line L790 (20.5752, -2.3854) -> (20.5933, -2.4016)
  line L791 (20.5933, -2.4016) -> (20.6154, -2.418)
  line L792 (20.6154, -2.418) -> (20.6414, -2.4345)
  line L793 (20.6414, -2.4345) -> (20.7182, -2.4748)
  line L794 (20.7182, -2.4748) -> (20.7708, -2.5043)
  line L795 (20.7708, -2.5043) -> (20.8376, -2.5457)
  line L796 (20.8376, -2.5457) -> (20.9117, -2.5959)
  line L797 (20.9117, -2.5959) -> (20.9951, -2.6578)
  line L798 (20.9951, -2.6578) -> (21.0858, -2.731)
  line L799 (21.0858, -2.731) -> (21.1838, -2.8172)
  line L800 (21.1838, -2.8172) -> (21.2886, -2.9175)
  line L801 (21.2886, -2.9175) -> (21.3426, -2.9724)
  line L802 (21.3426, -2.9724) -> (21.4406, -3.0783)
  arc A21 (21.3021, -3.4243) -> (21.4406, -3.0783) centre (13.25, 0) ccw
  line L803 (21.3021, -3.4243) -> (21.1581, -3.4333)
  line L804 (21.1581, -3.4333) -> (21.0811, -3.4358)
  line L805 (21.0811, -3.4358) -> (20.9361, -3.4361)
  line L806 (20.9361, -3.4361) -> (20.8057, -3.4308)
  line L807 (20.8057, -3.4308) -> (20.6895, -3.4212)
  line L808 (20.6895, -3.4212) -> (20.5864, -3.4084)
  line L809 (20.5864, -3.4084) -> (20.4981, -3.3937)
  line L810 (20.4981, -3.3937) -> (20.4212, -3.3775)
  line L811 (20.4212, -3.3775) -> (20.3628, -3.3626)
  line L812 (20.3628, -3.3626) -> (20.2794, -3.3387)
  line L813 (20.2794, -3.3387) -> (20.2492, -3.3327)
  line L814 (20.2492, -3.3327) -> (20.2219, -3.3294)
  line L815 (20.2219, -3.3294) -> (20.1976, -3.3286)
  line L816 (20.1976, -3.3286) -> (20.1763, -3.3302)
  line L817 (20.1763, -3.3302) -> (20.1582, -3.3341)
  line L818 (20.1582, -3.3341) -> (20.1434, -3.3401)
  line L819 (20.1434, -3.3401) -> (20.1318, -3.3482)
  line L820 (20.1318, -3.3482) -> (20.1237, -3.3581)
  line L821 (20.1237, -3.3581) -> (20.113, -3.3797)
  line L822 (20.113, -3.3797) -> (20.0496, -3.5054)
  line L823 (20.0496, -3.5054) -> (19.9839, -3.63)
  line L824 (19.9839, -3.63) -> (19.9726, -3.6512)
  line L825 (19.9726, -3.6512) -> (19.9692, -3.6636)
  line L826 (19.9692, -3.6636) -> (19.9693, -3.6777)
  line L827 (19.9693, -3.6777) -> (19.973, -3.6933)
  line L828 (19.973, -3.6933) -> (19.9803, -3.7103)
  line L829 (19.9803, -3.7103) -> (19.9914, -3.7286)
  line L830 (19.9914, -3.7286) -> (20.0061, -3.7479)
  line L831 (20.0061, -3.7479) -> (20.0247, -3.7682)
  line L832 (20.0247, -3.7682) -> (20.0471, -3.7893)
  line L833 (20.0471, -3.7893) -> (20.1149, -3.8434)
  line L834 (20.1149, -3.8434) -> (20.1609, -3.8824)
  line L835 (20.1609, -3.8824) -> (20.2187, -3.9356)
  line L836 (20.2187, -3.9356) -> (20.2819, -3.999)
  line L837 (20.2819, -3.999) -> (20.3522, -4.0755)
  line L838 (20.3522, -4.0755) -> (20.4273, -4.1646)
  line L839 (20.4273, -4.1646) -> (20.5073, -4.2678)
  line L840 (20.5073, -4.2678) -> (20.5912, -4.3861)
  line L841 (20.5912, -4.3861) -> (20.6338, -4.4502)
  line L842 (20.6338, -4.4502) -> (20.7101, -4.5727)
  arc A22 (20.5085, -4.8863) -> (20.7101, -4.5727) centre (13.25, 0) ccw
  line L843 (20.5085, -4.8863) -> (20.3654, -4.8679)
  line L844 (20.3654, -4.8679) -> (20.2894, -4.8558)
  line L845 (20.2894, -4.8558) -> (20.1469, -4.8286)
  line L846 (20.1469, -4.8286) -> (20.0198, -4.7987)
  line L847 (20.0198, -4.7987) -> (19.9076, -4.7673)
  line L848 (19.9076, -4.7673) -> (19.8088, -4.7352)
  line L849 (19.8088, -4.7352) -> (19.7249, -4.7041)
  line L850 (19.7249, -4.7041) -> (19.6525, -4.6736)
  line L851 (19.6525, -4.6736) -> (19.5979, -4.6479)
  line L852 (19.5979, -4.6479) -> (19.5205, -4.6087)
  line L853 (19.5205, -4.6087) -> (19.492, -4.5971)
  line L854 (19.492, -4.5971) -> (19.4658, -4.5886)
  line L855 (19.4658, -4.5886) -> (19.4421, -4.5832)
  line L856 (19.4421, -4.5832) -> (19.4209, -4.5808)
  line L857 (19.4209, -4.5808) -> (19.4024, -4.5812)
  line L858 (19.4024, -4.5812) -> (19.3867, -4.5843)
  line L859 (19.3867, -4.5843) -> (19.3738, -4.5901)
  line L860 (19.3738, -4.5901) -> (19.3639, -4.5983)
  line L861 (19.3639, -4.5983) -> (19.3493, -4.6175)
  line L862 (19.3493, -4.6175) -> (19.2633, -4.7289)
  line L863 (19.2633, -4.7289) -> (19.1753, -4.8388)
  line L864 (19.1753, -4.8388) -> (19.1601, -4.8575)
  line L865 (19.1601, -4.8575) -> (19.1544, -4.869)
  line L866 (19.1544, -4.869) -> (19.1519, -4.8829)
  line L867 (19.1519, -4.8829) -> (19.1525, -4.8989)
  line L868 (19.1525, -4.8989) -> (19.1565, -4.917)
  line L869 (19.1565, -4.917) -> (19.1639, -4.937)
  line L870 (19.1639, -4.937) -> (19.1747, -4.9588)
  line L871 (19.1747, -4.9588) -> (19.1891, -4.9822)
  line L872 (19.1891, -4.9822) -> (19.2071, -5.0072)
  line L873 (19.2071, -5.0072) -> (19.2635, -5.0732)
  line L874 (19.2635, -5.0732) -> (19.3013, -5.1201)
  line L875 (19.3013, -5.1201) -> (19.348, -5.1833)
  line L876 (19.348, -5.1833) -> (19.3981, -5.2575)
  line L877 (19.3981, -5.2575) -> (19.4525, -5.3459)
  line L878 (19.4525, -5.3459) -> (19.5095, -5.4477)
  line L879 (19.5095, -5.4477) -> (19.5685, -5.5641)
  line L880 (19.5685, -5.5641) -> (19.6285, -5.6961)
  line L881 (19.6285, -5.6961) -> (19.6582, -5.7672)
  line L882 (19.6582, -5.7672) -> (19.7098, -5.9019)
  arc A23 (19.4526, -6.1717) -> (19.7098, -5.9019) centre (13.25, 0) ccw
  line L883 (19.4526, -6.1717) -> (19.3156, -6.1265)
  line L884 (19.3156, -6.1265) -> (19.2432, -6.1002)
  line L885 (19.2432, -6.1002) -> (19.1084, -6.0465)
  line L886 (19.1084, -6.0465) -> (18.9893, -5.9932)
  line L887 (18.9893, -5.9932) -> (18.885, -5.9411)
  line L888 (18.885, -5.9411) -> (18.7941, -5.8909)
  line L889 (18.7941, -5.8909) -> (18.7176, -5.8444)
  line L890 (18.7176, -5.8444) -> (18.6523, -5.8008)
  line L891 (18.6523, -5.8008) -> (18.6036, -5.7653)
  line L892 (18.6036, -5.7653) -> (18.5349, -5.7121)
  line L893 (18.5349, -5.7121) -> (18.5092, -5.6953)
  line L894 (18.5092, -5.6953) -> (18.4851, -5.6821)
  line L895 (18.4851, -5.6821) -> (18.4628, -5.6723)
  line L896 (18.4628, -5.6723) -> (18.4425, -5.6659)
  line L897 (18.4425, -5.6659) -> (18.4242, -5.6628)
  line L898 (18.4242, -5.6628) -> (18.4082, -5.6629)
  line L899 (18.4082, -5.6629) -> (18.3945, -5.6661)
  line L900 (18.3945, -5.6661) -> (18.3832, -5.6723)
  line L901 (18.3832, -5.6723) -> (18.3653, -5.6883)
  line L902 (18.3653, -5.6883) -> (18.2597, -5.7815)
  line L903 (18.2597, -5.7815) -> (18.1524, -5.8727)
  line L904 (18.1524, -5.8727) -> (18.134, -5.8882)
  line L905 (18.134, -5.8882) -> (18.1262, -5.8985)
  line L906 (18.1262, -5.8985) -> (18.1211, -5.9116)
  line L907 (18.1211, -5.9116) -> (18.1188, -5.9275)
  line L908 (18.1188, -5.9275) -> (18.1192, -5.946)
  line L909 (18.1192, -5.946) -> (18.1227, -5.967)
  line L910 (18.1227, -5.967) -> (18.1292, -5.9904)
  line L911 (18.1292, -5.9904) -> (18.1389, -6.0162)
  line L912 (18.1389, -6.0162) -> (18.1518, -6.0441)
  line L913 (18.1518, -6.0441) -> (18.1947, -6.1196)
  line L914 (18.1947, -6.1196) -> (18.2229, -6.1728)
  line L915 (18.2229, -6.1728) -> (18.2568, -6.2437)
  line L916 (18.2568, -6.2437) -> (18.292, -6.326)
  line L917 (18.292, -6.326) -> (18.3287, -6.4232)
  line L918 (18.3287, -6.4232) -> (18.3654, -6.5338)
  line L919 (18.3654, -6.5338) -> (18.4013, -6.6593)
  line L920 (18.4013, -6.6593) -> (18.4352, -6.8003)
  line L921 (18.4352, -6.8003) -> (18.4509, -6.8757)
  line L922 (18.4509, -6.8757) -> (18.4762, -7.0178)
  arc A24 (18.1725, -7.234) -> (18.4762, -7.0178) centre (13.25, 0) ccw
  line L923 (18.1725, -7.234) -> (18.0465, -7.1637)
  line L924 (18.0465, -7.1637) -> (17.9804, -7.1242)
  line L925 (17.9804, -7.1242) -> (17.8583, -7.046)
  line L926 (17.8583, -7.046) -> (17.7514, -6.9711)
  line L927 (17.7514, -6.9711) -> (17.6588, -6.9002)
  line L928 (17.6588, -6.9002) -> (17.5791, -6.8337)
  line L929 (17.5791, -6.8337) -> (17.5128, -6.7736)
  line L930 (17.5128, -6.7736) -> (17.4568, -6.7184)
  line L931 (17.4568, -6.7184) -> (17.4157, -6.6742)
  line L932 (17.4157, -6.6742) -> (17.3584, -6.6091)
  line L933 (17.3584, -6.6091) -> (17.3363, -6.5877)
  line L934 (17.3363, -6.5877) -> (17.3151, -6.5701)
  line L935 (17.3151, -6.5701) -> (17.2951, -6.5563)
  line L936 (17.2951, -6.5563) -> (17.2764, -6.5462)
  line L937 (17.2764, -6.5462) -> (17.259, -6.5397)
  line L938 (17.259, -6.5397) -> (17.2433, -6.5367)
  line L939 (17.2433, -6.5367) -> (17.2292, -6.5373)
  line L940 (17.2292, -6.5373) -> (17.217, -6.5412)
  line L941 (17.217, -6.5412) -> (17.1963, -6.5536)
  line L942 (17.1963, -6.5536) -> (17.075, -6.6251)
  line L943 (17.075, -6.6251) -> (16.9524, -6.6944)